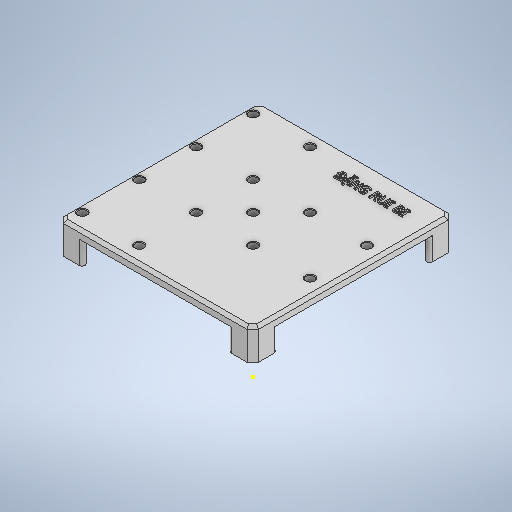
# Autodesk Inventor part: Repick
Saved by Autodesk Inventor 2025 (Build 290162000, 162)
## iProperties
Created: 2026-07-17
Part Number: Repick
Material: Generic
Document SubType Name: Sheet Metal
Designer: MSI
Density: 1 g/cm^3
Sheet Metal Rule: Default_mm
Appearance: Default
Author: MSI
Autodesk Inventor part; units mm, degrees
ref_plane "YZ Plane" through (0, 0, 0) normal (1, 0, 0) x (0, 1, 0)
ref_plane "XZ Plane" through (0, 0, 0) normal (0, 1, 0) x (-1, 0, 0)
ref_plane "XY Plane" through (0, 0, 0) normal (0, 0, 1) x (1, 0, 0)
sketch "Sketch1" plane through (0, 0, 0) normal (0, 1, 0) x (-1, 0, 0)
  circle A0 centre (80, -20) radius 1.5
  circle A1 centre (80, -40) radius 1.5
  circle A2 centre (80, -60) radius 1.5
  circle A3 centre (80, -80) radius 1.5
  circle A4 centre (60, -80) radius 1.5
  circle A5 centre (60, -60) radius 1.5
  circle A6 centre (60, -40) radius 1.5
  circle A7 centre (60, -20) radius 1.5
  circle A8 centre (20, -60) radius 1.5
  circle A9 centre (20, -40) radius 1.5
  circle A10 centre (40, -60) radius 1.5
  circle A11 centre (40, -40) radius 1.5
  circle A12 centre (50, -50) radius 1.5
  line L0 (82.9894, -14.3145) -> (14.4573, -14.3145)
  line L1 (14.4573, -14.3145) -> (14.4573, -84.9883)
  line L2 (14.4573, -84.9883) -> (82.9894, -84.9883)
  line L3 (82.9894, -84.9883) -> (82.9894, -14.3145)
  point P0 (0, 0)
  dimension "d4" = 3
  dimension "d5" = 3
  dimension "d6" = 3
  dimension "d7" = 3
  dimension "d8" = 3
  dimension "d9" = 3
  dimension "d10" = 3
  dimension "d11" = 3
  dimension "d13" = 3
  dimension "d14" = 3
  dimension "d15" = 3
  dimension "d16" = 3
  dimension "d17" = 60
  dimension "d20" = 3
  constraints: 13 centre point, 8 end point, 2 parallel, 1 horizontal, 1 perpendicular
  measures "d4" diameter of A0
  measures "d5" diameter of A1
  measures "d6" diameter of A2
  measures "d7" diameter of A3
  measures "d8" diameter of A4
  measures "d9" diameter of A5
  measures "d10" diameter of A6
  measures "d11" diameter of A7
  measures "d13" diameter of A8
  measures "d14" diameter of A9
  measures "d15" diameter of A10
  measures "d16" diameter of A11
  measures "d17" distance of A3.centre A0.centre
  measures "d20" diameter of A12
extrude "Extrusion1" add sketch "Sketch1" along normal blind 3
chamfer "Chamfer1" distance 2 angle 45 4 edges at (-14.4573, 1.5, -14.3145) (-14.4573, 1.5, -84.9883) (-82.9894, 1.5, -84.9883) (-82.9894, 1.5, -14.3145)
sketch "Sketch2" plane through (0, 0, 0) normal (0, -1, 0) x (1, 0, 0)
  line L0 (-14.4573, -16.3145) -> (-14.4573, -82.9883) projected
  line L1 (-14.4573, -82.9883) -> (-14.4573, -74.9883)
  line L2 (-16.4573, -84.9883) -> (-80.9894, -84.9883) projected
  line L3 (-16.4573, -84.9883) -> (-24.4573, -84.9883)
  line L4 (-24.4573, -84.9883) -> (-14.4573, -74.9883)
  line L5 (-16.4573, -84.9883) -> (-14.4573, -82.9883) projected
  line L6 (-16.4573, -84.9883) -> (-14.4573, -82.9883)
  line L7 (-80.9894, -84.9883) -> (-72.9894, -84.9883)
  line L8 (-82.9894, -82.9883) -> (-82.9894, -16.3145) projected
  line L9 (-80.9894, -84.9883) -> (-82.9894, -82.9883)
  line L10 (-82.9894, -82.9883) -> (-82.9894, -74.9883)
  line L11 (-82.9894, -74.9883) -> (-72.9894, -84.9883)
  line L12 (-80.9894, -14.3145) -> (-16.4573, -14.3145) projected
  line L13 (-16.4573, -14.3145) -> (-24.4573, -14.3145)
  line L14 (-16.4573, -14.3145) -> (-14.4573, -16.3145)
  line L15 (-14.4573, -16.3145) -> (-14.4573, -24.3145)
  line L16 (-14.4573, -24.3145) -> (-24.4573, -14.3145)
  line L17 (-82.9894, -16.3145) -> (-82.9894, -24.3145)
  line L18 (-82.9894, -16.3145) -> (-80.9894, -14.3145)
  line L19 (-80.9894, -14.3145) -> (-72.9894, -14.3145)
  line L20 (-72.9894, -14.3145) -> (-82.9894, -24.3145)
  point P0 (0, 0)
  dimension "d26" = 8
  dimension "d27" = 8
  dimension "d28" = 8
  dimension "d29" = 8
  dimension "d30" = 8
  dimension "d31" = 8
  dimension "d32" = 8
  dimension "d33" = 8
  constraints: 32 end point, 8 point on line, 1 collinear
  measures "d26" distance of L0.end L1.end
  measures "d27" distance of L2.start L3.end
  measures "d28" distance of L2.end L7.end
  measures "d29" distance of L8.start L10.end
  measures "d30" distance of L12.end L13.end
  measures "d31" distance of L0.start L15.end
  measures "d32" distance of L8.end L17.end
  measures "d33" distance of L12.start L19.end
extrude "Extrusion2" add sketch "Sketch2" along normal blind 8 contours L0 L16 L12 L14 | L0 L5 L2 L4 | L20 L8 L18 L12 | L2 L9 L8 L11
extrude "Extrusion3" cut sketch "Sketch1" against normal blind 3 contours A0 | A3
fillet "Fillet1" radius 1 1 edges at (-82.9894, -4, -24.3145)
fillet "Fillet2" radius 1 7 edges at (-72.9894, -4, -14.3145) (-14.4573, -4, -24.3145) (-14.4573, -4, -74.9883) (-24.4573, -4, -84.9883) (-72.9894, -4, -84.9883) (-24.4573, -4, -14.3145) (-82.9894, -4, -74.9883)
chamfer "Chamfer2" distance 0.2 angle 45 13 edges at (-78.5, 3, -80) (-58.5, 3, -80) (-58.5, 3, -60) (-78.5, 3, -60) (-38.5, 3, -60) (-18.5, 3, -60) (-18.5, 3, -40) (-38.5, 3, -40) (-48.5, 3, -50) (-58.5, 3, -40) (-58.5, 3, -20) (-78.5, 3, -40) (-78.5, 3, -20)
chamfer "Chamfer3" distance 1 angle 45 8 edges at (-48.7233, 3, -14.3145) (-14.4573, 3, -49.6514) (-48.7233, 3, -84.9883) (-82.9894, 3, -49.6514) (-81.9894, 3, -83.9883) (-15.4573, 3, -83.9883) (-15.4573, 3, -15.3145) (-81.9894, 3, -15.3145)
sketch "Sketch3" plane through (0, 3, 0) normal (0, 1, 0) x (1, 0, 0)
  line L0 (-46.7777, 78.8211) -> (-22.9577, 78.8211) construction
  line L1 (-22.9577, 78.8211) -> (-22.9577, 69.2931) construction
  line L2 (-22.9577, 69.2931) -> (-46.7777, 69.2931) construction
  line L3 (-46.7777, 69.2931) -> (-46.7777, 78.8211) construction
  spline S0 degree 2 poles (-43.9816, 76.23) (-43.9816, 75.8126) (-44.32, 75.1408) (-44.6041, 74.953) knots 0 0 0 1 2 2 2
  spline S1 degree 2 poles (-44.6041, 74.953) (-44.8313, 74.7999) (-45.313, 74.7085) (-45.6835, 74.7085) knots 0 0 0 1 2 2 2
  line L4 (-45.6835, 74.7085) -> (-46.3849, 74.7085)
  line L5 (-46.3849, 74.7085) -> (-46.3849, 76.2251)
  line L6 (-46.3849, 76.2251) -> (-46.7283, 76.2251)
  line L7 (-46.7283, 76.2251) -> (-46.7283, 76.5166)
  line L8 (-46.7283, 76.5166) -> (-46.3849, 76.5166)
  line L9 (-46.3849, 76.5166) -> (-46.3849, 77.7565)
  line L10 (-46.3849, 77.7565) -> (-45.6909, 77.7565)
  spline S2 degree 2 poles (-45.6909, 77.7565) (-45.2611, 77.7565) (-44.772, 77.6281) (-44.5991, 77.5145) knots 0 0 0 1 2 2 2
  spline S3 degree 2 poles (-44.5991, 77.5145) (-44.3052, 77.3193) (-43.9816, 76.6746) (-43.9816, 76.23) knots 0 0 0 1 2 2 2
  spline S4 degree 2 poles (-44.404, 76.235) (-44.404, 76.5857) (-44.6362, 77.0822) (-44.8659, 77.223) knots 0 0 0 1 2 2 2
  spline S5 degree 2 poles (-44.8659, 77.223) (-45.0289, 77.3193) (-45.3969, 77.4058) (-45.6711, 77.4058) knots 0 0 0 1 2 2 2
  line L11 (-45.6711, 77.4058) -> (-45.9799, 77.4058)
  line L12 (-45.9799, 77.4058) -> (-45.9799, 76.5166)
  line L13 (-45.9799, 76.5166) -> (-45.3105, 76.5166)
  line L14 (-45.3105, 76.5166) -> (-45.3105, 76.2251)
  line L15 (-45.3105, 76.2251) -> (-45.9799, 76.2251)
  line L16 (-45.9799, 76.2251) -> (-45.9799, 75.0593)
  line L17 (-45.9799, 75.0593) -> (-45.6711, 75.0593)
  spline S6 degree 2 poles (-45.6711, 75.0593) (-45.4019, 75.0593) (-44.9943, 75.1482) (-44.8288, 75.2618) knots 0 0 0 1 2 2 2
  spline S7 degree 2 poles (-44.8288, 75.2618) (-44.6164, 75.4051) (-44.404, 75.8793) (-44.404, 76.235) knots 0 0 0 1 2 2 2
  line L18 (-43.8705, 74.7085) -> (-42.8429, 77.7565)
  line L19 (-42.8429, 77.7565) -> (-42.344, 77.7565)
  line L20 (-42.344, 77.7565) -> (-41.3165, 74.7085)
  line L21 (-41.3165, 74.7085) -> (-41.7438, 74.7085)
  line L22 (-41.7438, 74.7085) -> (-42.0204, 75.5607)
  line L23 (-42.0204, 75.5607) -> (-43.1838, 75.5607)
  line L24 (-43.1838, 75.5607) -> (-43.4604, 74.7085)
  line L25 (-43.4604, 74.7085) -> (-43.8705, 74.7085)
  line L26 (-42.1316, 75.9065) -> (-42.6034, 77.3415)
  line L27 (-42.6034, 77.3415) -> (-43.0727, 75.9065)
  line L28 (-43.0727, 75.9065) -> (-42.1316, 75.9065)
  spline S8 degree 2 poles (-41.9192, 78.8211) (-41.9192, 78.6457) (-42.0056, 78.3567) (-42.0846, 78.2579) knots 0 0 0 1 2 2 2
  spline S9 degree 2 poles (-42.0846, 78.2579) (-42.176, 78.1492) (-42.4107, 78.0406) (-42.5935, 78.0406) knots 0 0 0 1 2 2 2
  spline S10 degree 2 poles (-42.5935, 78.0406) (-42.7614, 78.0406) (-43.0109, 78.1542) (-43.0974, 78.2579) knots 0 0 0 1 2 2 2
  spline S11 degree 2 poles (-43.0974, 78.2579) (-43.1813, 78.3592) (-43.2678, 78.6482) (-43.2678, 78.8211) knots 0 0 0 1 2 2 2
  line L29 (-43.2678, 78.8211) -> (-42.9368, 78.8211)
  spline S12 degree 2 poles (-42.9368, 78.8211) (-42.9368, 78.5444) (-42.7639, 78.2999) (-42.5935, 78.2999) knots 0 0 0 1 2 2 2
  spline S13 degree 2 poles (-42.5935, 78.2999) (-42.4305, 78.2999) (-42.2501, 78.5395) (-42.2501, 78.8211) knots 0 0 0 1 2 2 2
  line L30 (-42.2501, 78.8211) -> (-41.9192, 78.8211)
  line L31 (-42.3687, 73.9255) -> (-42.8059, 73.9255)
  line L32 (-42.8059, 73.9255) -> (-42.8059, 74.3257)
  line L33 (-42.8059, 74.3257) -> (-42.3687, 74.3257)
  line L34 (-42.3687, 74.3257) -> (-42.3687, 73.9255)
  line L35 (-38.8465, 74.7085) -> (-39.3009, 74.7085)
  line L36 (-39.3009, 74.7085) -> (-40.6496, 77.3366)
  line L37 (-40.6496, 77.3366) -> (-40.6496, 74.7085)
  line L38 (-40.6496, 74.7085) -> (-41.0275, 74.7085)
  line L39 (-41.0275, 74.7085) -> (-41.0275, 77.7565)
  line L40 (-41.0275, 77.7565) -> (-40.452, 77.7565)
  line L41 (-40.452, 77.7565) -> (-39.2244, 75.3433)
  line L42 (-39.2244, 75.3433) -> (-39.2244, 77.7565)
  line L43 (-39.2244, 77.7565) -> (-38.8465, 77.7565)
  line L44 (-38.8465, 77.7565) -> (-38.8465, 74.7085)
  spline S14 degree 2 poles (-36.952, 74.6492) (-37.2755, 74.6492) (-37.8115, 74.8468) (-38.0042, 75.0469) knots 0 0 0 1 2 2 2
  spline S15 degree 2 poles (-38.0042, 75.0469) (-38.1968, 75.2494) (-38.4019, 75.8472) (-38.4019, 76.235) knots 0 0 0 1 2 2 2
  spline S16 degree 2 poles (-38.4019, 76.235) (-38.4019, 76.603) (-38.1944, 77.1859) (-38.0017, 77.3934) knots 0 0 0 1 2 2 2
  spline S17 degree 2 poles (-38.0017, 77.3934) (-37.8165, 77.5935) (-37.2731, 77.8109) (-36.9495, 77.8109) knots 0 0 0 1 2 2 2
  spline S18 degree 2 poles (-36.9495, 77.8109) (-36.7939, 77.8109) (-36.5123, 77.7664) (-36.3839, 77.7269) knots 0 0 0 1 2 2 2
  spline S19 degree 2 poles (-36.3839, 77.7269) (-36.2801, 77.6972) (-36.0282, 77.5886) (-35.9516, 77.549) knots 0 0 0 1 2 2 2
  line L45 (-35.9516, 77.549) -> (-35.9516, 77.06)
  line L46 (-35.9516, 77.06) -> (-35.9862, 77.06)
  spline S20 degree 2 poles (-35.9862, 77.06) (-36.0627, 77.1267) (-36.2233, 77.2477) (-36.3715, 77.3168) knots 0 0 0 1 2 2 2
  spline S21 degree 2 poles (-36.3715, 77.3168) (-36.495, 77.3786) (-36.8136, 77.4601) (-36.9964, 77.4601) knots 0 0 0 1 2 2 2
  spline S22 degree 2 poles (-36.9964, 77.4601) (-37.4361, 77.4601) (-37.9795, 76.7981) (-37.9795, 76.2473) knots 0 0 0 1 2 2 2
  spline S23 degree 2 poles (-37.9795, 76.2473) (-37.9795, 75.9411) (-37.8362, 75.4816) (-37.7004, 75.3235) knots 0 0 0 1 2 2 2
  spline S24 degree 2 poles (-37.7004, 75.3235) (-37.5695, 75.1655) (-37.199, 75) (-36.9668, 75) knots 0 0 0 1 2 2 2
  spline S25 degree 2 poles (-36.9668, 75) (-36.7963, 75) (-36.4555, 75.0494) (-36.3394, 75.0988) knots 0 0 0 1 2 2 2
  line L47 (-36.3394, 75.0988) -> (-36.3394, 75.8867)
  line L48 (-36.3394, 75.8867) -> (-37.0458, 75.8867)
  line L49 (-37.0458, 75.8867) -> (-37.0458, 76.2424)
  line L50 (-37.0458, 76.2424) -> (-35.9392, 76.2424)
  line L51 (-35.9392, 76.2424) -> (-35.9392, 74.9111)
  spline S26 degree 2 poles (-35.9392, 74.9111) (-36.0158, 74.8765) (-36.2776, 74.7703) (-36.3888, 74.7382) knots 0 0 0 1 2 2 2
  spline S27 degree 2 poles (-36.3888, 74.7382) (-36.5395, 74.6937) (-36.7815, 74.6492) (-36.952, 74.6492) knots 0 0 0 1 2 2 2
  line L52 (-31.7625, 74.7085) -> (-32.2886, 74.7085)
  line L53 (-32.2886, 74.7085) -> (-33.2519, 75.9213)
  line L54 (-33.2519, 75.9213) -> (-33.7162, 75.9213)
  line L55 (-33.7162, 75.9213) -> (-33.7162, 74.7085)
  line L56 (-33.7162, 74.7085) -> (-34.1213, 74.7085)
  line L57 (-34.1213, 74.7085) -> (-34.1213, 77.7565)
  line L58 (-34.1213, 77.7565) -> (-33.3359, 77.7565)
  spline S28 degree 2 poles (-33.3359, 77.7565) (-33.074, 77.7565) (-32.7208, 77.6997) (-32.5603, 77.596) knots 0 0 0 1 2 2 2
  spline S29 degree 2 poles (-32.5603, 77.596) (-32.3997, 77.4922) (-32.2145, 77.1686) (-32.2145, 76.9291) knots 0 0 0 1 2 2 2
  spline S30 degree 2 poles (-32.2145, 76.9291) (-32.2145, 76.5956) (-32.5553, 76.1436) (-32.8468, 76.0349) knots 0 0 0 1 2 2 2
  line L59 (-32.8468, 76.0349) -> (-31.7625, 74.7085)
  spline S31 degree 2 poles (-32.6368, 76.8969) (-32.6368, 77.0303) (-32.7307, 77.2353) (-32.8295, 77.302) knots 0 0 0 1 2 2 2
  spline S32 degree 2 poles (-32.8295, 77.302) (-32.9159, 77.3588) (-33.1457, 77.4058) (-33.3136, 77.4058) knots 0 0 0 1 2 2 2
  line L60 (-33.3136, 77.4058) -> (-33.7162, 77.4058)
  line L61 (-33.7162, 77.4058) -> (-33.7162, 76.2597)
  line L62 (-33.7162, 76.2597) -> (-33.3606, 76.2597)
  spline S33 degree 2 poles (-33.3606, 76.2597) (-33.1852, 76.2597) (-32.9061, 76.3214) (-32.8097, 76.4178) knots 0 0 0 1 2 2 2
  spline S34 degree 2 poles (-32.8097, 76.4178) (-32.7208, 76.5017) (-32.6368, 76.7389) (-32.6368, 76.8969) knots 0 0 0 1 2 2 2
  spline S35 degree 2 poles (-30.4558, 74.6443) (-30.725, 74.6443) (-31.1252, 74.7851) (-31.266, 74.9259) knots 0 0 0 1 2 2 2
  spline S36 degree 2 poles (-31.266, 74.9259) (-31.4265, 75.084) (-31.5574, 75.5286) (-31.5574, 75.8546) knots 0 0 0 1 2 2 2
  line L63 (-31.5574, 75.8546) -> (-31.5574, 77.7565)
  line L64 (-31.5574, 77.7565) -> (-31.1524, 77.7565)
  line L65 (-31.1524, 77.7565) -> (-31.1524, 75.8546)
  spline S37 degree 2 poles (-31.1524, 75.8546) (-31.1524, 75.6422) (-31.098, 75.3557) (-31.0214, 75.2396) knots 0 0 0 1 2 2 2
  spline S38 degree 2 poles (-31.0214, 75.2396) (-30.9399, 75.1161) (-30.6584, 74.9901) (-30.4558, 74.9901) knots 0 0 0 1 2 2 2
  spline S39 degree 2 poles (-30.4558, 74.9901) (-30.2656, 74.9901) (-29.9692, 75.1161) (-29.8877, 75.2396) knots 0 0 0 1 2 2 2
  spline S40 degree 2 poles (-29.8877, 75.2396) (-29.8111, 75.3557) (-29.7568, 75.6397) (-29.7568, 75.8447) knots 0 0 0 1 2 2 2
  line L66 (-29.7568, 75.8447) -> (-29.7568, 77.7565)
  line L67 (-29.7568, 77.7565) -> (-29.3517, 77.7565)
  line L68 (-29.3517, 77.7565) -> (-29.3517, 75.8546)
  spline S41 degree 2 poles (-29.3517, 75.8546) (-29.3517, 75.536) (-29.4802, 75.0815) (-29.6432, 74.9259) knots 0 0 0 1 2 2 2
  spline S42 degree 2 poles (-29.6432, 74.9259) (-29.7889, 74.7826) (-30.1742, 74.6443) (-30.4558, 74.6443) knots 0 0 0 1 2 2 2
  line L69 (-27.7092, 74.7085) -> (-28.8898, 74.7085)
  line L70 (-28.8898, 74.7085) -> (-28.8898, 75.0197)
  line L71 (-28.8898, 75.0197) -> (-28.502, 75.0197)
  line L72 (-28.502, 75.0197) -> (-28.502, 77.4453)
  line L73 (-28.502, 77.4453) -> (-28.8898, 77.4453)
  line L74 (-28.8898, 77.4453) -> (-28.8898, 77.7565)
  line L75 (-28.8898, 77.7565) -> (-27.7092, 77.7565)
  line L76 (-27.7092, 77.7565) -> (-27.7092, 77.4453)
  line L77 (-27.7092, 77.4453) -> (-28.0969, 77.4453)
  line L78 (-28.0969, 77.4453) -> (-28.0969, 75.0197)
  line L79 (-28.0969, 75.0197) -> (-27.7092, 75.0197)
  line L80 (-27.7092, 75.0197) -> (-27.7092, 74.7085)
  spline S43 degree 2 poles (-23.8312, 75.6446) (-23.8312, 75.4174) (-24.0041, 75.0691) (-24.1474, 74.9555) knots 0 0 0 1 2 2 2
  spline S44 degree 2 poles (-24.1474, 74.9555) (-24.3203, 74.8221) (-24.713, 74.7085) (-25.0242, 74.7085) knots 0 0 0 1 2 2 2
  line L81 (-25.0242, 74.7085) -> (-25.8986, 74.7085)
  line L82 (-25.8986, 74.7085) -> (-25.8986, 77.7565)
  line L83 (-25.8986, 77.7565) -> (-25.0909, 77.7565)
  spline S45 degree 2 poles (-25.0909, 77.7565) (-24.7649, 77.7565) (-24.4389, 77.7145) (-24.2907, 77.633) knots 0 0 0 1 2 2 2
  spline S46 degree 2 poles (-24.2907, 77.633) (-24.1252, 77.5466) (-23.9745, 77.2625) (-23.9745, 77.0698) knots 0 0 0 1 2 2 2
  spline S47 degree 2 poles (-23.9745, 77.0698) (-23.9745, 76.855) (-24.2017, 76.5141) (-24.4018, 76.4178) knots 0 0 0 1 2 2 2
  line L84 (-24.4018, 76.4178) -> (-24.4018, 76.4029)
  spline S48 degree 2 poles (-24.4018, 76.4029) (-24.1301, 76.3288) (-23.8312, 75.9361) (-23.8312, 75.6446) knots 0 0 0 1 2 2 2
  spline S49 degree 2 poles (-24.2536, 75.6274) (-24.2536, 75.8003) (-24.3524, 76.0226) (-24.5006, 76.1016) knots 0 0 0 1 2 2 2
  spline S50 degree 2 poles (-24.5006, 76.1016) (-24.5969, 76.151) (-24.8242, 76.1806) (-25.0341, 76.1806) knots 0 0 0 1 2 2 2
  line L85 (-25.0341, 76.1806) -> (-25.4935, 76.1806)
  line L86 (-25.4935, 76.1806) -> (-25.4935, 75.0543)
  line L87 (-25.4935, 75.0543) -> (-25.165, 75.0543)
  spline S51 degree 2 poles (-25.165, 75.0543) (-24.8983, 75.0543) (-24.592, 75.1037) (-24.4734, 75.1828) knots 0 0 0 1 2 2 2
  spline S52 degree 2 poles (-24.4734, 75.1828) (-24.3598, 75.2643) (-24.2536, 75.4668) (-24.2536, 75.6274) knots 0 0 0 1 2 2 2
  spline S53 degree 2 poles (-24.3969, 77.013) (-24.3969, 77.1217) (-24.471, 77.2847) (-24.5525, 77.3317) knots 0 0 0 1 2 2 2
  spline S54 degree 2 poles (-24.5525, 77.3317) (-24.6513, 77.386) (-24.8909, 77.4107) (-25.1058, 77.4107) knots 0 0 0 1 2 2 2
  line L88 (-25.1058, 77.4107) -> (-25.4935, 77.4107)
  line L89 (-25.4935, 77.4107) -> (-25.4935, 76.519)
  line L90 (-25.4935, 76.519) -> (-25.0341, 76.519)
  spline S55 degree 2 poles (-25.0341, 76.519) (-24.8439, 76.519) (-24.6636, 76.5586) (-24.5673, 76.6203) knots 0 0 0 1 2 2 2
  spline S56 degree 2 poles (-24.5673, 76.6203) (-24.4734, 76.6796) (-24.3969, 76.8698) (-24.3969, 77.013) knots 0 0 0 1 2 2 2
  line L91 (-22.3665, 74.7085) -> (-23.5472, 74.7085)
  line L92 (-23.5472, 74.7085) -> (-23.5472, 75.0197)
  line L93 (-23.5472, 75.0197) -> (-23.1594, 75.0197)
  line L94 (-23.1594, 75.0197) -> (-23.1594, 77.4453)
  line L95 (-23.1594, 77.4453) -> (-23.5472, 77.4453)
  line L96 (-23.5472, 77.4453) -> (-23.5472, 77.7565)
  line L97 (-23.5472, 77.7565) -> (-22.3665, 77.7565)
  line L98 (-22.3665, 77.7565) -> (-22.3665, 77.4453)
  line L99 (-22.3665, 77.4453) -> (-22.7543, 77.4453)
  line L100 (-22.7543, 77.4453) -> (-22.7543, 75.0197)
  line L101 (-22.7543, 75.0197) -> (-22.3665, 75.0197)
  line L102 (-22.3665, 75.0197) -> (-22.3665, 74.7085)
  point P0 (0, 0)
  constraints: 2 other
extrude "Extrusion4" add sketch "Sketch3" along normal blind 0.5
sketch "Sketch4" plane through (0, 3, 0) normal (0, 1, 0) x (1, 0, 0)
  point P0 (0, 0)
equation "\"BendRadius\" = Thickness"
equation "\"BendReliefWidth\" = Thickness"
equation "\"BendReliefDepth\" = 0.5 * Thickness"
equation "\"CornerReliefSize\" = 4 * Thickness"
equation "\"MinimumRemnant\" = 2 * Thickness"
equation "\"TransitionRadius\" = BendRadius"
equation "\"JacobiRadiusSize\" = BendRadius"
equation "\"GapSize\" = Thickness"
equation "\"Thickness\" = 0.5"
body "Solid1"
